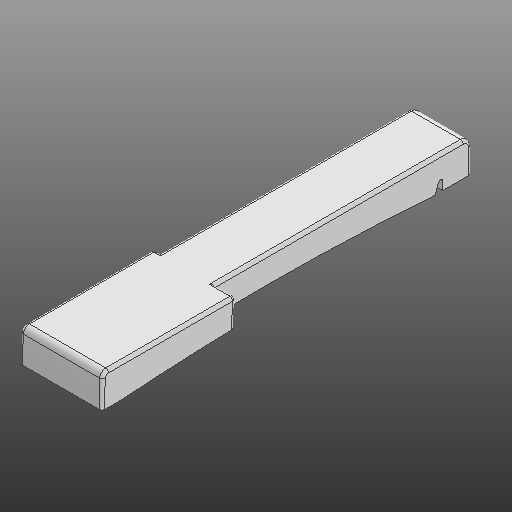
# Autodesk Inventor part: GKey0
Saved by Autodesk Inventor 2020 (Build 240168000, 168)
## iProperties
Created: 2019-12-01
Part Number: GKey0
Material: Generic
Document SubType Name: Modeling
Designer: Isaac Newcomb
Density: 1 g/cm^3
Appearance: Default
Mass: 10.4551 g
Surface Area: 47.4511 cm^2
Volume: 10.4551 cm^3
Project: Ice Keys
slotOffset: 1.174 mm
hingeRad: 0.500 mm
upperWidth: 6.700 mm
my_slotHeadOffset: 1.000 mm
my_slotHeadHeight: 3.000 mm
my_slotHeadWidth: 6.200 mm
my_neckSlotWidth: 4.300 mm
my_edgeSoftenRad: 0.700 mm
my_backWidth: 7.000 mm
my_hingeDepth: 2.000 mm
my_hingeCutRad: 0.550 mm
uRight: 6.700 mm
Author: Isaac Newcomb
Autodesk Inventor part; units mm, degrees
ref_plane "YZ Plane" through (0, 0, 0) normal (1, 0, 0) x (0, 1, 0)
ref_plane "XZ Plane" through (0, 0, 0) normal (0, 1, 0) x (-1, 0, 0)
ref_plane "Slot Start Plane" through (0, 0, -1.7245) normal (0, 0, 1) x (1, 0, 0)
sketch "Key Profile" plane through (0, 0, 0) normal (1, 0, 0) x (0, 1, 0)
  line L0 (-2, 2.8563) -> (0.684, 1.8794)
  arc A0 (1.6188, -1.1745) -> (0.684, 1.8794) centre (0, 0) ccw
  line L1 (-2, 1.3132) -> (0.1881, 0.5168)
  arc A1 (0, -0.55) -> (0.1881, 0.5168) centre (0, 0) ccw
  line L2 (-2, 2.8563) -> (-2, -0.55)
  line L3 (0, 0) -> (-2, 0) construction
  line L4 (0, -0.55) -> (-2, -0.55)
  line L5 (1.6188, -1.1745) -> (-0.097, -0.55)
  line L6 (6, -5.55) -> (6, 87.7952)
  line L7 (-2, 87.9773) -> (-2, 2.8563)
  arc A2 (6, 87.7952) -> (-2, 87.9773) centre (0, 0) ccw
  line L8 (-2, -0.55) -> (-2, -7.55)
  arc A3 (4, -7.55) -> (6, -5.55) centre (4, -5.55) ccw
  line L9 (-2, -7.55) -> (4, -7.55)
  arc A4 (6, 55.1747) -> (-2, 55.464) centre (0, 0) ccw
  arc A5 (-2, 2.8563) -> (-2, 83.2148) centre (-539.3737, 43.0355) ccw
  point P0 (-0.5, 43.0355)
  point P1 (-0.6441, 55.4963)
  dimension "my_hingeCutRad" = 0.55
  dimension "my_hingeDepth" = 2
  dimension "my_hingeRegCutRad" = 2
  dimension "keyLength" = 88
  dimension "my_KeyHeight" = 8
  dimension "d107" = 20
  dimension "d122" = 4
  dimension "slotOffset" = 1.1745
  dimension "my_backWidth" = 7
  dimension "d128" = 55.5
  dimension "d135" = 1.5
  dimension "d136" = 4.7625
  constraints: 21 end point, 14 point on circle, 6 centre point, 6 point on line, 6 tangent, 4 coincident, 3 horizontal, 3 parallel, 2 vertical, 1 collinear
  measures "my_hingeCutRad" radius of A1
  measures "my_hingeDepth" distance of L3.start L3.end
  measures "my_hingeRegCutRad" radius of A0
  measures "keyLength" radius of A2
  measures "my_KeyHeight" distance from line of L6.start L7
  measures "d107" angle of L4 L1
  measures "d122" horizontal distance of A0.centre L9.end
  measures "slotOffset" vertical distance of L5.start point (0, 0)
  measures "my_backWidth" distance of L2.end L8.end
  measures "d128" radius of A4
  measures "d135" distance from line of L7 point (-0.5, 43.036)
  measures "d136" distance of L7.start A5.end
extrude "Upper (u)" add sketch "Key Profile" along normal blind 6.7 and the other way blind 6.7 contours A5 A4 L6 A3 L9 L8 L4 L5 A0 L0 | L0 A0 L5 L4 A1 L1 L2
extrude "Lower (d)" add sketch "Key Profile" along normal blind 11.75 and the other way blind 8.3214 contours A5 L7 A2 L6 A4
extrude "Protrusion Cutout" cut sketch "Key Profile" along normal mid plane 4.5 contours L0 A0 L5 L4 A1 L1 L2
fillet "Front Fillet" radius 1.5 1 edges at (1.7143, 6, 87.7952)
sketch "Slot Sketch" plane through (0, 0, -1.7245) normal (0, 0, 1) x (1, 0, 0)
  line L0 (2.15, -2) -> (2.15, 1)
  line L1 (3.1, 4) -> (-3.1, 4)
  line L2 (-2.15, 1) -> (-2.15, -2)
  line L3 (-2.15, -2) -> (2.15, -2)
  line L4 (0, -2) -> (0, 4) construction
  line L5 (-3.1, 4) -> (-3.1, 1)
  line L6 (-3.1, 1) -> (-2.15, 1)
  line L7 (2.15, 1) -> (3.1, 1)
  line L8 (3.1, 1) -> (3.1, 4)
  point P0 (0, 0)
  dimension "d109" = 2
  dimension "my_slotHeadOffset" = 1
  dimension "my_slotHeadHeight" = 3
  dimension "my_slotHeadWidth" = 6.2
  dimension "my_neckSlotWidth" = 4.3
  constraints: 18 end point, 4 perpendicular, 3 parallel, 2 midpoint, 2 point on line, 2 vertical
  measures "d109" distance from line of point (0, 0) L3
  measures "my_slotHeadOffset" distance from line of L6 point (0, 0)
  measures "my_slotHeadHeight" distance of L1.end L5.end
  measures "my_slotHeadWidth" distance of L1.start L1.end
  measures "my_neckSlotWidth" distance of L2.end L0.start
extrude "Slot" cut sketch "Slot Sketch" against normal through all
fillet "Edge Softening" radius 0.7 16 edges at (6.7, 5.4142, -6.9642) (6.7, 1, -7.55) (6.7, 6, 24.8124) (-6.7, 5.4142, -6.9642) (-6.7, 1, -7.55) (-6.7, 6, 24.8124) (-8.3214, 5.5879, 87.4156) (-8.3214, 1.2899, 87.9905) (-8.3214, 6, 70.7788) (11.75, 5.5879, 87.4156) (11.75, 1.2899, 87.9905) (11.75, 6, 70.7788) (-8.3214, 2.6828, 55.4351) (11.75, 2.6828, 55.4351) (9.225, 6, 55.1747) (-7.5107, 6, 55.1747)
equation "\"my_headHeight\" = 3"
equation "\"my_headOffset\" = 1"
equation "\"whiteKeyWidth\" = 20.07143"
body "Solid1"
